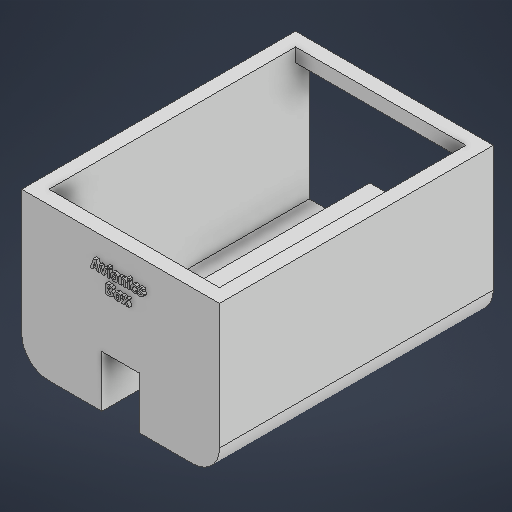
# Autodesk Inventor part: Avionics_Box
Saved by Autodesk Inventor 2027 (Build 310192060, 192F)
## iProperties
Created: 2026-06-08
Part Number: Avionics_Box
Material: Generic
Document SubType Name: Modeling
Designer: rbilo
Density: 1 g/cm^3
Appearance: Default
Author: rbilo
Autodesk Inventor part; units mm, degrees
ref_plane "YZ Plane" through (0, 0, 0) normal (1, 0, 0) x (0, 1, 0)
ref_plane "XZ Plane" through (0, 0, 0) normal (0, 1, 0) x (-1, 0, 0)
ref_plane "XY Plane" through (0, 0, 0) normal (0, 0, 1) x (1, 0, 0)
sketch "Sketch1" plane through (0, 0, 0) normal (0, 1, 0) x (-1, 0, 0)
  line L0 (-65, 90) -> (65, 90)
  line L1 (65, 90) -> (65, -90)
  line L2 (65, -90) -> (-65, -90)
  line L3 (-65, -90) -> (-65, 90)
  line L4 (-65, 90) -> (65, -90) construction
  line L5 (65, 90) -> (-65, -90) construction
  point P0 (0, 0)
  dimension "d0" = 180
  dimension "d1" = 130
  constraints: 12 end point, 2 midpoint, 2 parallel, 1 horizontal, 1 perpendicular
  measures "d0" distance of L1.end L0.end
  measures "d1" distance of L0.start L0.end
extrude "Extrusion1" add sketch "Sketch1" along normal blind 100
sketch "Sketch2" plane through (-65, 0, 90) normal (0, 0, 1) x (1, 0, 0)
  line L0 (52.75, -34) -> (77.25, -34)
  line L1 (77.25, -34) -> (77.25, 34)
  line L2 (77.25, 34) -> (52.75, 34)
  line L3 (52.75, 34) -> (52.75, -34)
  line L4 (52.75, -34) -> (77.25, 34) construction
  line L5 (77.25, -34) -> (52.75, 34) construction
  line L6 (0, 0) -> (130, 0) projected
  point P0 (65, 0)
  point P1 (65, 34)
  dimension "d4" = 24.5
  dimension "d5" = 34
  constraints: 12 end point, 3 midpoint, 2 parallel, 1 horizontal, 1 perpendicular
  measures "d4" distance between parallel lines of L1 L3
  measures "d5" distance from line of point (65, 34) L6
extrude "Extrusion2" cut sketch "Sketch2" against normal blind 180
shell "Shell1" thickness 9 removed faces 0
sketch "Sketch3" plane through (0, 100, 0) normal (0, 1, 0) x (1, 0, 0)
  line L0 (-56, -81) -> (56, -81)
  line L1 (56, -81) -> (56, 81)
  line L2 (56, 81) -> (-56, 81)
  line L3 (-56, 81) -> (-56, -81)
  line L4 (-56, -81) -> (56, 81) construction
  line L5 (56, -81) -> (-56, 81) construction
  line L6 (65, 90) -> (-65, 90) projected
  line L7 (-65, 90) -> (-65, -90) projected
  point P0 (0, 0)
  dimension "d9" = 9
  dimension "d10" = 9
  constraints: 12 end point, 2 midpoint, 2 parallel, 1 horizontal, 1 perpendicular
  measures "d9" distance between parallel lines of L6 L2
  measures "d10" distance between parallel lines of L7 L3
extrude "Extrusion3" cut sketch "Sketch3" against normal blind 9
sketch "Sketch5" plane through (-65, 100, 90) normal (0, 0, 1) x (1, 0, 0)
  line L0 (51.2267, -13.6211) -> (77.9251, -13.6211) construction
  line L1 (77.9251, -13.6211) -> (77.9251, -16.879) construction
  line L2 (77.9251, -16.879) -> (51.2267, -16.879) construction
  line L3 (51.2267, -16.879) -> (51.2267, -13.6211) construction
  line L4 (47.0907, -19.9937) -> (49.1506, -13.8977)
  line L5 (49.1506, -13.8977) -> (50.8204, -13.8977)
  line L6 (50.8204, -13.8977) -> (52.8804, -19.9937)
  line L7 (52.8804, -19.9937) -> (51.3045, -19.9937)
  line L8 (51.3045, -19.9937) -> (50.9241, -18.7488)
  line L9 (50.9241, -18.7488) -> (49.0074, -18.7488)
  line L10 (49.0074, -18.7488) -> (48.6221, -19.9937)
  line L11 (48.6221, -19.9937) -> (47.0907, -19.9937)
  line L12 (50.5882, -17.6423) -> (49.9658, -15.6267)
  line L13 (49.9658, -15.6267) -> (49.3384, -17.6423)
  line L14 (49.3384, -17.6423) -> (50.5882, -17.6423)
  line L15 (57.7068, -15.3946) -> (56.0568, -19.9937)
  line L16 (56.0568, -19.9937) -> (54.4908, -19.9937)
  line L17 (54.4908, -19.9937) -> (52.8557, -15.3946)
  line L18 (52.8557, -15.3946) -> (54.3624, -15.3946)
  line L19 (54.3624, -15.3946) -> (55.3059, -18.4327)
  line L20 (55.3059, -18.4327) -> (56.2297, -15.3946)
  line L21 (56.2297, -15.3946) -> (57.7068, -15.3946)
  line L22 (59.6877, -19.9937) -> (58.2551, -19.9937)
  line L23 (58.2551, -19.9937) -> (58.2551, -15.3946)
  line L24 (58.2551, -15.3946) -> (59.6877, -15.3946)
  line L25 (59.6877, -15.3946) -> (59.6877, -19.9937)
  line L26 (59.7322, -14.7375) -> (58.2156, -14.7375)
  line L27 (58.2156, -14.7375) -> (58.2156, -13.6211)
  line L28 (58.2156, -13.6211) -> (59.7322, -13.6211)
  line L29 (59.7322, -13.6211) -> (59.7322, -14.7375)
  spline S0 degree 2 poles (65.1959, -17.6966) (65.1959, -18.8328) (63.9559, -20.137) (62.8247, -20.137) knots 0 0 0 1 2 2 2
  spline S1 degree 2 poles (62.8247, -20.137) (61.6983, -20.137) (60.4485, -18.8328) (60.4485, -17.6966) knots 0 0 0 1 2 2 2
  spline S2 degree 2 poles (60.4485, -17.6966) (60.4485, -16.5505) (61.6983, -15.2513) (62.8247, -15.2513) knots 0 0 0 1 2 2 2
  spline S3 degree 2 poles (62.8247, -15.2513) (63.951, -15.2513) (65.1959, -16.5555) (65.1959, -17.6966) knots 0 0 0 1 2 2 2
  spline S4 degree 2 poles (63.7287, -17.7065) (63.7287, -17.2965) (63.5953, -16.7481) (63.4767, -16.5851) knots 0 0 0 1 2 2 2
  spline S5 degree 2 poles (63.4767, -16.5851) (63.3483, -16.4122) (63.0272, -16.2788) (62.8247, -16.2788) knots 0 0 0 1 2 2 2
  spline S6 degree 2 poles (62.8247, -16.2788) (62.6271, -16.2788) (62.3158, -16.3974) (62.1874, -16.5653) knots 0 0 0 1 2 2 2
  spline S7 degree 2 poles (62.1874, -16.5653) (62.0639, -16.7234) (61.9157, -17.2816) (61.9157, -17.7065) knots 0 0 0 1 2 2 2
  spline S8 degree 2 poles (61.9157, -17.7065) (61.9157, -18.1264) (62.054, -18.6451) (62.1676, -18.8032) knots 0 0 0 1 2 2 2
  spline S9 degree 2 poles (62.1676, -18.8032) (62.2813, -18.9613) (62.6271, -19.1095) (62.8345, -19.1095) knots 0 0 0 1 2 2 2
  spline S10 degree 2 poles (62.8345, -19.1095) (63.0074, -19.1095) (63.3631, -18.9613) (63.4718, -18.8131) knots 0 0 0 1 2 2 2
  spline S11 degree 2 poles (63.4718, -18.8131) (63.5953, -18.6402) (63.7287, -18.1412) (63.7287, -17.7065) knots 0 0 0 1 2 2 2
  line L30 (70.2594, -19.9937) -> (68.8169, -19.9937)
  line L31 (68.8169, -19.9937) -> (68.8169, -17.7164)
  spline S12 degree 2 poles (68.8169, -17.7164) (68.8169, -17.4348) (68.7725, -16.8815) (68.7132, -16.7531) knots 0 0 0 1 2 2 2
  spline S13 degree 2 poles (68.7132, -16.7531) (68.6391, -16.595) (68.3624, -16.4616) (68.1253, -16.4616) knots 0 0 0 1 2 2 2
  spline S14 degree 2 poles (68.1253, -16.4616) (67.9524, -16.4616) (67.5918, -16.595) (67.3892, -16.7382) knots 0 0 0 1 2 2 2
  line L32 (67.3892, -16.7382) -> (67.3892, -19.9937)
  line L33 (67.3892, -19.9937) -> (65.9566, -19.9937)
  line L34 (65.9566, -19.9937) -> (65.9566, -15.3946)
  line L35 (65.9566, -15.3946) -> (67.3892, -15.3946)
  line L36 (67.3892, -15.3946) -> (67.3892, -15.9034)
  spline S15 degree 2 poles (67.3892, -15.9034) (67.74, -15.607) (68.4069, -15.2711) (68.812, -15.2711) knots 0 0 0 1 2 2 2
  spline S16 degree 2 poles (68.812, -15.2711) (69.5135, -15.2711) (70.2594, -16.1603) (70.2594, -17.0001) knots 0 0 0 1 2 2 2
  line L37 (70.2594, -17.0001) -> (70.2594, -19.9937)
  line L38 (72.7541, -19.9937) -> (71.3215, -19.9937)
  line L39 (71.3215, -19.9937) -> (71.3215, -15.3946)
  line L40 (71.3215, -15.3946) -> (72.7541, -15.3946)
  line L41 (72.7541, -15.3946) -> (72.7541, -19.9937)
  line L42 (72.7986, -14.7375) -> (71.282, -14.7375)
  line L43 (71.282, -14.7375) -> (71.282, -13.6211)
  line L44 (71.282, -13.6211) -> (72.7986, -13.6211)
  line L45 (72.7986, -13.6211) -> (72.7986, -14.7375)
  spline S17 degree 2 poles (76.1035, -20.1172) (75.5354, -20.1172) (74.5918, -19.8307) (74.2411, -19.5343) knots 0 0 0 1 2 2 2
  spline S18 degree 2 poles (74.2411, -19.5343) (73.9002, -19.233) (73.5149, -18.3289) (73.5149, -17.7164) knots 0 0 0 1 2 2 2
  spline S19 degree 2 poles (73.5149, -17.7164) (73.5149, -17.0544) (73.9298, -16.1306) (74.2905, -15.8342) knots 0 0 0 1 2 2 2
  spline S20 degree 2 poles (74.2905, -15.8342) (74.6313, -15.5477) (75.5601, -15.2711) (76.0639, -15.2711) knots 0 0 0 1 2 2 2
  spline S21 degree 2 poles (76.0639, -15.2711) (76.4443, -15.2711) (77.2051, -15.4489) (77.5904, -15.6416) knots 0 0 0 1 2 2 2
  line L46 (77.5904, -15.6416) -> (77.5904, -16.8667)
  line L47 (77.5904, -16.8667) -> (77.4076, -16.8667)
  spline S22 degree 2 poles (77.4076, -16.8667) (77.3187, -16.7827) (77.0717, -16.5851) (76.9235, -16.5061) knots 0 0 0 1 2 2 2
  spline S23 degree 2 poles (76.9235, -16.5061) (76.7654, -16.4171) (76.3752, -16.2986) (76.1331, -16.2986) knots 0 0 0 1 2 2 2
  spline S24 degree 2 poles (76.1331, -16.2986) (75.5848, -16.2986) (74.9821, -17.0643) (74.9821, -17.7164) knots 0 0 0 1 2 2 2
  spline S25 degree 2 poles (74.9821, -17.7164) (74.9821, -18.408) (75.6243, -19.0897) (76.1578, -19.0897) knots 0 0 0 1 2 2 2
  spline S26 degree 2 poles (76.1578, -19.0897) (76.4295, -19.0897) (76.8346, -18.9662) (76.9828, -18.8773) knots 0 0 0 1 2 2 2
  spline S27 degree 2 poles (76.9828, -18.8773) (77.126, -18.7933) (77.3335, -18.6056) (77.4076, -18.5315) knots 0 0 0 1 2 2 2
  line L48 (77.4076, -18.5315) -> (77.5904, -18.5315)
  line L49 (77.5904, -18.5315) -> (77.5904, -19.7615)
  spline S28 degree 2 poles (77.5904, -19.7615) (77.4669, -19.8159) (77.1458, -19.9542) (76.9778, -19.9987) knots 0 0 0 1 2 2 2
  spline S29 degree 2 poles (76.9778, -19.9987) (76.7704, -20.0579) (76.4048, -20.1172) (76.1035, -20.1172) knots 0 0 0 1 2 2 2
  spline S30 degree 2 poles (79.6702, -20.1172) (79.1663, -20.1172) (78.2623, -19.8949) (77.9659, -19.7467) knots 0 0 0 1 2 2 2
  line L50 (77.9659, -19.7467) -> (77.9659, -18.5364)
  line L51 (77.9659, -18.5364) -> (78.0844, -18.5364)
  spline S31 degree 2 poles (78.0844, -18.5364) (78.1882, -18.6155) (78.45, -18.8032) (78.6822, -18.9069) knots 0 0 0 1 2 2 2
  spline S32 degree 2 poles (78.6822, -18.9069) (78.8847, -19.0008) (79.3836, -19.1342) (79.68, -19.1342) knots 0 0 0 1 2 2 2
  spline S33 degree 2 poles (79.68, -19.1342) (79.9814, -19.1342) (80.4458, -18.9464) (80.4458, -18.7439) knots 0 0 0 1 2 2 2
  spline S34 degree 2 poles (80.4458, -18.7439) (80.4458, -18.5858) (80.2333, -18.4179) (79.927, -18.3487) knots 0 0 0 1 2 2 2
  spline S35 degree 2 poles (79.927, -18.3487) (79.764, -18.3042) (79.2651, -18.2104) (79.0724, -18.1511) knots 0 0 0 1 2 2 2
  spline S36 degree 2 poles (79.0724, -18.1511) (78.529, -17.9831) (77.9856, -17.3261) (77.9856, -16.7876) knots 0 0 0 1 2 2 2
  spline S37 degree 2 poles (77.9856, -16.7876) (77.9856, -16.4814) (78.2672, -15.938) (78.5438, -15.7255) knots 0 0 0 1 2 2 2
  spline S38 degree 2 poles (78.5438, -15.7255) (78.8155, -15.5181) (79.6208, -15.2711) (80.1296, -15.2711) knots 0 0 0 1 2 2 2
  spline S39 degree 2 poles (80.1296, -15.2711) (80.6137, -15.2711) (81.4239, -15.4637) (81.7005, -15.5971) knots 0 0 0 1 2 2 2
  line L52 (81.7005, -15.5971) -> (81.7005, -16.7629)
  line L53 (81.7005, -16.7629) -> (81.5869, -16.7629)
  spline S40 degree 2 poles (81.5869, -16.7629) (81.5128, -16.7037) (81.1917, -16.511) (81.0435, -16.4418) knots 0 0 0 1 2 2 2
  spline S41 degree 2 poles (81.0435, -16.4418) (80.8607, -16.3628) (80.4161, -16.2541) (80.1839, -16.2541) knots 0 0 0 1 2 2 2
  spline S42 degree 2 poles (80.1839, -16.2541) (79.8727, -16.2541) (79.4429, -16.4665) (79.4429, -16.6394) knots 0 0 0 1 2 2 2
  spline S43 degree 2 poles (79.4429, -16.6394) (79.4429, -16.7975) (79.6553, -16.9754) (80.011, -17.0643) knots 0 0 0 1 2 2 2
  spline S44 degree 2 poles (80.011, -17.0643) (80.1938, -17.1087) (80.673, -17.1927) (80.8953, -17.2668) knots 0 0 0 1 2 2 2
  spline S45 degree 2 poles (80.8953, -17.2668) (81.3893, -17.4249) (81.9031, -18.0424) (81.9031, -18.5562) knots 0 0 0 1 2 2 2
  spline S46 degree 2 poles (81.9031, -18.5562) (81.9031, -18.8773) (81.6017, -19.4651) (81.3201, -19.6627) knots 0 0 0 1 2 2 2
  spline S47 degree 2 poles (81.3201, -19.6627) (81.0287, -19.8801) (80.2284, -20.1172) (79.6702, -20.1172) knots 0 0 0 1 2 2 2
  spline S48 degree 2 poles (62.0688, -28.1633) (62.0688, -28.6178) (61.723, -29.3044) (61.4365, -29.5317) knots 0 0 0 1 2 2 2
  spline S49 degree 2 poles (61.4365, -29.5317) (61.0907, -29.8034) (60.2707, -30.0306) (59.6334, -30.0306) knots 0 0 0 1 2 2 2
  line L54 (59.6334, -30.0306) -> (57.198, -30.0306)
  line L55 (57.198, -30.0306) -> (57.198, -23.9346)
  line L56 (57.198, -23.9346) -> (59.3469, -23.9346)
  spline S50 degree 2 poles (59.3469, -23.9346) (60.0187, -23.9346) (60.7103, -24.0384) (61.0117, -24.2014) knots 0 0 0 1 2 2 2
  spline S51 degree 2 poles (61.0117, -24.2014) (61.3426, -24.3743) (61.6637, -24.9671) (61.6637, -25.3524) knots 0 0 0 1 2 2 2
  spline S52 degree 2 poles (61.6637, -25.3524) (61.6637, -25.797) (61.2191, -26.4936) (60.8239, -26.6566) knots 0 0 0 1 2 2 2
  line L57 (60.8239, -26.6566) -> (60.8239, -26.6862)
  spline S53 degree 2 poles (60.8239, -26.6862) (61.392, -26.8048) (62.0688, -27.5409) (62.0688, -28.1633) knots 0 0 0 1 2 2 2
  spline S54 degree 2 poles (60.488, -28.1386) (60.488, -27.8521) (60.2608, -27.531) (60.0335, -27.447) knots 0 0 0 1 2 2 2
  spline S55 degree 2 poles (60.0335, -27.447) (59.8952, -27.3927) (59.4062, -27.3828) (59.0011, -27.3828) knots 0 0 0 1 2 2 2
  line L58 (59.0011, -27.3828) -> (58.7195, -27.3828)
  line L59 (58.7195, -27.3828) -> (58.7195, -28.9191)
  line L60 (58.7195, -28.9191) -> (58.8035, -28.9191)
  spline S56 degree 2 poles (58.8035, -28.9191) (59.3963, -28.9191) (59.8508, -28.9043) (60.0879, -28.8006) knots 0 0 0 1 2 2 2
  spline S57 degree 2 poles (60.0879, -28.8006) (60.2954, -28.7067) (60.488, -28.3609) (60.488, -28.1386) knots 0 0 0 1 2 2 2
  spline S58 degree 2 poles (60.1076, -25.6538) (60.1076, -25.5056) (59.9545, -25.1943) (59.7964, -25.1252) knots 0 0 0 1 2 2 2
  spline S59 degree 2 poles (59.7964, -25.1252) (59.6482, -25.056) (59.2333, -25.0461) (58.8232, -25.0461) knots 0 0 0 1 2 2 2
  line L61 (58.8232, -25.0461) -> (58.7195, -25.0461)
  line L62 (58.7195, -25.0461) -> (58.7195, -26.3404)
  line L63 (58.7195, -26.3404) -> (58.9121, -26.3404)
  spline S60 degree 2 poles (58.9121, -26.3404) (59.3024, -26.3404) (59.6186, -26.3256) (59.7865, -26.2466) knots 0 0 0 1 2 2 2
  spline S61 degree 2 poles (59.7865, -26.2466) (59.9693, -26.1576) (60.1076, -25.8563) (60.1076, -25.6538) knots 0 0 0 1 2 2 2
  spline S62 degree 2 poles (67.2756, -27.7335) (67.2756, -28.8697) (66.0357, -30.1739) (64.9044, -30.1739) knots 0 0 0 1 2 2 2
  spline S63 degree 2 poles (64.9044, -30.1739) (63.7781, -30.1739) (62.5283, -28.8697) (62.5283, -27.7335) knots 0 0 0 1 2 2 2
  spline S64 degree 2 poles (62.5283, -27.7335) (62.5283, -26.5874) (63.7781, -25.2882) (64.9044, -25.2882) knots 0 0 0 1 2 2 2
  spline S65 degree 2 poles (64.9044, -25.2882) (66.0307, -25.2882) (67.2756, -26.5924) (67.2756, -27.7335) knots 0 0 0 1 2 2 2
  spline S66 degree 2 poles (65.8084, -27.7434) (65.8084, -27.3334) (65.6751, -26.785) (65.5565, -26.622) knots 0 0 0 1 2 2 2
  spline S67 degree 2 poles (65.5565, -26.622) (65.4281, -26.4491) (65.107, -26.3157) (64.9044, -26.3157) knots 0 0 0 1 2 2 2
  spline S68 degree 2 poles (64.9044, -26.3157) (64.7068, -26.3157) (64.3956, -26.4343) (64.2671, -26.6022) knots 0 0 0 1 2 2 2
  spline S69 degree 2 poles (64.2671, -26.6022) (64.1436, -26.7603) (63.9954, -27.3186) (63.9954, -27.7434) knots 0 0 0 1 2 2 2
  spline S70 degree 2 poles (63.9954, -27.7434) (63.9954, -28.1633) (64.1338, -28.682) (64.2474, -28.8401) knots 0 0 0 1 2 2 2
  spline S71 degree 2 poles (64.2474, -28.8401) (64.361, -28.9982) (64.7068, -29.1464) (64.9143, -29.1464) knots 0 0 0 1 2 2 2
  spline S72 degree 2 poles (64.9143, -29.1464) (65.0872, -29.1464) (65.4429, -28.9982) (65.5516, -28.85) knots 0 0 0 1 2 2 2
  spline S73 degree 2 poles (65.5516, -28.85) (65.6751, -28.6771) (65.8084, -28.1781) (65.8084, -27.7434) knots 0 0 0 1 2 2 2
  line L64 (72.5713, -30.0306) -> (70.8917, -30.0306)
  line L65 (70.8917, -30.0306) -> (70.0173, -28.7116)
  line L66 (70.0173, -28.7116) -> (69.1183, -30.0306)
  line L67 (69.1183, -30.0306) -> (67.4732, -30.0306)
  line L68 (67.4732, -30.0306) -> (69.1677, -27.7286)
  line L69 (69.1677, -27.7286) -> (67.5029, -25.4315)
  line L70 (67.5029, -25.4315) -> (69.1825, -25.4315)
  line L71 (69.1825, -25.4315) -> (70.042, -26.7257)
  line L72 (70.042, -26.7257) -> (70.9065, -25.4315)
  line L73 (70.9065, -25.4315) -> (72.5516, -25.4315)
  line L74 (72.5516, -25.4315) -> (70.8868, -27.694)
  line L75 (70.8868, -27.694) -> (72.5713, -30.0306)
  point P0 (65, -100)
  constraints: 2 other
extrude "Extrusion5" add sketch "Sketch5" along normal blind 2
sketch "Sketch6" plane through (-65, 100, 90) normal (0, 0, 1) x (1, 0, 0)
  line L0 (0, -100) -> (0, -82.3223)
  line L1 (0, -100) -> (0, 0) projected
  line L2 (0, -100) -> (17.6777, -100)
  line L3 (52.75, -100) -> (0, -100) projected
  line L4 (0, -100) -> (17.6777, -82.3223) construction
  arc A0 (0, -82.3223) -> (17.6777, -100) centre (17.6777, -82.3223) ccw
  point P0 (65, -100)
  dimension "d23" = 17.6777
  dimension "d24" = 17.6777
  constraints: 6 end point, 2 point on circle, 2 point on line, 1 centre point, 1 coincident
  measures "d23" distance of L0.start L0.end
  measures "d24" distance of L0.start L2.end
extrude "Extrusion6" cut sketch "Sketch6" against normal blind 180
sketch "Sketch7" plane through (-65, 100, 90) normal (0, 0, 1) x (1, 0, 0)
  line L0 (130, -100) -> (130, -82.3223)
  line L1 (130, -100) -> (112.3223, -100)
  line L2 (130, -100) -> (130, -78.0983)
  line L3 (130, -100) -> (130, -82.8406)
  line L4 (77.25, -100) -> (130, -100) projected
  line L5 (130, -100) -> (112.3223, -82.3223) construction
  arc A0 (112.3223, -100) -> (130, -82.3223) centre (112.3223, -82.3223) ccw
  point P0 (65, -100)
  dimension "d27" = 17.6777
  dimension "d28" = 17.6777
  dimension "d29" = 17.6777
  dimension "d30" = 17.6777
  constraints: 10 end point, 2 point on circle, 1 centre point, 1 coincident, 1 horizontal, 1 point on line
  measures "d27" distance of L0.start L1.end
  measures "d28" distance of L0.start L0.end
  measures "d29" horizontal distance of L0.start L5.end
  measures "d30" horizontal distance of L0.start L5.end
extrude "Extrusion7" cut sketch "Sketch7" against normal blind 180
sketch "Sketch8" plane through (65, 100, -90) normal (0, 0, -1) x (-1, 0, 0)
  line L0 (9, -9) -> (121, -9)
  line L1 (121, -9) -> (121, -62)
  line L2 (121, -62) -> (9, -62)
  line L3 (9, -62) -> (9, -9)
  line L4 (9, -62) -> (48.75, -62)
  line L5 (48.75, -62) -> (48.75, -91)
  line L6 (48.75, -91) -> (9, -91)
  line L7 (9, -91) -> (9, -62)
  line L8 (121, -62) -> (81.25, -62)
  line L9 (81.25, -62) -> (81.25, -91)
  line L10 (81.25, -91) -> (121, -91)
  line L11 (121, -91) -> (121, -62)
  line L12 (77.25, -100) -> (112.3223, -100) projected
  line L13 (130, -82.3223) -> (130, 0) projected
  line L14 (0, -82.3223) -> (0, 0) projected
  line L15 (52.75, -100) -> (52.75, -66) projected
  line L16 (77.25, -66) -> (77.25, -100) projected
  line L17 (52.75, -66) -> (77.25, -66) projected
  line L18 (0, 0) -> (130, 0) projected
  point P0 (65, -100)
  dimension "d34" = 9
  dimension "d35" = 9
  dimension "d36" = 9
  dimension "d37" = 4
  dimension "d38" = 4
  dimension "d39" = 4
  dimension "d40" = 9
  constraints: 24 end point, 6 parallel, 3 horizontal, 3 perpendicular, 1 point on line
  measures "d34" distance between parallel lines of L12 L10
  measures "d35" distance between parallel lines of L13 L11
  measures "d36" distance between parallel lines of L14 L7
  measures "d37" distance between parallel lines of L15 L5
  measures "d38" distance between parallel lines of L9 L16
  measures "d39" distance between parallel lines of L17 L2
  measures "d40" distance between parallel lines of L18 L0
extrude "Extrusion8" cut sketch "Sketch8" against normal blind 171
sketch "Sketch9" plane through (0, 0, 0) normal (0, -1, 0) x (1, 0, 0)
  line L0 (12.25, 90) -> (12.25, -90) projected
  line L1 (12.25, 90) -> (47.3223, 90) construction
  line L2 (12.25, 90) -> (47.3223, 90)
  line L3 (29.7862, 90) -> (29.7862, -90) construction
  line L4 (56, -90) -> (-56, -90) construction
  line L5 (40.7604, 0) -> (40.7604, -90) construction
  line L6 (-56, -81) -> (56, -81) construction
  line L7 (40.7604, -45) -> (29.7862, -45) construction
  line L8 (40.7604, 0) -> (40.7604, 90) construction
  line L9 (40.7604, 45) -> (29.7862, 45) construction
  circle A0 centre (29.7862, 45) radius 3.18
  circle A1 centre (29.7862, -45) radius 3.175
  line L10 (-47.3223, -90) -> (-47.3223, 90) construction
  line L11 (-47.3223, 90) -> (-12.25, 90) projected
  line L12 (-47.3223, 90) -> (-12.25, 90) construction
  line L13 (-29.7862, 90) -> (-29.7862, -90) construction
  line L14 (-47.3223, 0) -> (-47.3223, -90) construction
  line L15 (-47.3223, -45) -> (-29.7862, -45) construction
  line L16 (-47.3223, 90) -> (-47.3223, 0) construction
  line L17 (-47.3223, 45) -> (-29.7862, 45) construction
  circle A2 centre (-29.7862, 45) radius 3.175
  circle A3 centre (-29.7862, -45) radius 3.175
  point P0 (0, 0)
  dimension "d43" = 6.36
  dimension "d44" = 6.35
  dimension "d45" = 6.35
  dimension "d46" = 6.35
  constraints: 24 end point, 8 perpendicular, 7 midpoint, 7 point on line, 4 centre point, 4 coincident, 3 collinear, 1 vertical
  measures "d43" diameter of A0
  measures "d44" diameter of A1
  measures "d45" diameter of A2
  measures "d46" diameter of A3
extrude "Extrusion9" cut sketch "Sketch9" against normal blind 9
body "Solid1"
